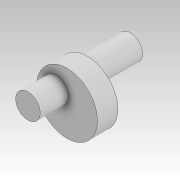
# Autodesk Inventor part: Camshaft
Saved by Autodesk Inventor 2020 (Build 240168000, 168)
## iProperties
Created: 2021-07-13
Part Number: Camshaft
Material: Generic
Document SubType Name: Modeling
Designer: DDeGo
Density: 1 g/cm^3
Appearance: Default
Author: DDeGo
Autodesk Inventor part; units mm, degrees
ref_plane "YZ Plane" through (0, 0, 0) normal (1, 0, 0) x (0, 1, 0)
ref_plane "XZ Plane" through (0, 0, 0) normal (0, 1, 0) x (-1, 0, 0)
ref_plane "XY Plane" through (0, 0, 0) normal (0, 0, 1) x (1, 0, 0)
derived "LiquidPistonMasterSketch.ipt"
sketch "CamshaftBearingID" plane through (6.645, 6.5847, 6.5) normal (0, 0, 1) x (1, 0, 0)
  circle A0 centre (-4.5125, -7.8159) radius 5.95
  point P0 (-6.645, -6.5847)
ref_plane "BotRotorCavity" through (0, 0, 2) normal (0, 0, 1) x (1, 0, 0)
ref_plane "TopRotorCavity" through (0, 0, 12) normal (0, 0, 1) x (1, 0, 0)
ref_plane "GearsTop" through (0, 0, 5) normal (0, 0, 1) x (1, 0, 0)
ref_plane "RotorCross" through (2.1325, -1.2312, 2) normal (0.8660254, -0.5, 0) x (0.5, 0.8660254, 0)
ref_plane "BearingCamBotID" through (6.645, 6.5847, 6.5) normal (0, 0, 1) x (1, 0, 0)
sketch "CamshaftPillar" plane through (0, 0, 2) normal (0.5, 0.8660254, 0) x (-0.8660254, 0.5, 0)
  line L0 (0, 14) -> (-2.4, 14)
  line L1 (-2.4, 14) -> (-2.4, -6)
  line L2 (-2.4, -6) -> (0, -6)
  line L3 (0, -6) -> (0, 14)
  line L4 (-7.3624, -2) -> (0, -2) construction
  point P0 (-2.4624, 10)
ref_plane "Midplane" through (0, 0, 2) normal (0.5, 0.8660254, 0) x (-0.8660254, 0.5, 0)
extrude "Extrusion1" add sketch "CamshaftBearingID" along normal blind 4
revolve "Revolution1" add sketch "CamshaftPillar" angle 360 about axis through (0, 0, -4) along (0, 0, 1)
ref_plane "Work Plane6" through (6.645, 6.5847, 6) normal (0, 0, 1) x (1, 0, 0)
body "Solid1"
